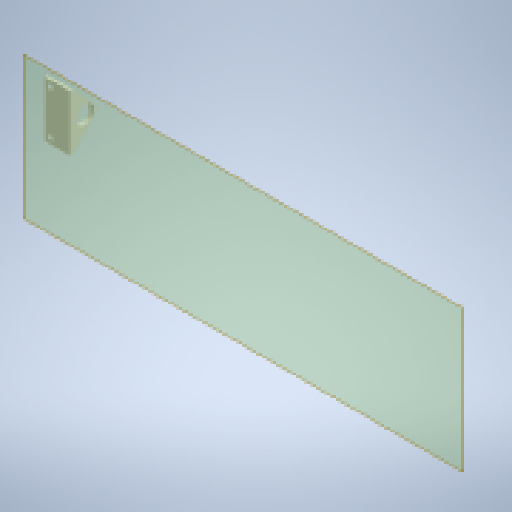
# Autodesk Inventor part: tumbler_holder
Saved by Autodesk Inventor 2024 (Build 280153000, 153)
## iProperties
Created: 2026-03-17
Part Number: tumbler_holder
Material: Generic
Document SubType Name: Modeling
Designer: SEMEN
Density: 1 g/cm^3
Appearance: Default
Author: SEMEN
Autodesk Inventor part; units mm, degrees
ref_plane "YZ Plane" through (0, 0, 0) normal (1, 0, 0) x (0, 1, 0)
ref_plane "XZ Plane" through (0, 0, 0) normal (0, 1, 0) x (-1, 0, 0)
ref_plane "XY Plane" through (0, 0, 0) normal (0, 0, 1) x (1, 0, 0)
ref_plane "Work Plane1" through (-14.6708, -27.7298, 48.581) normal (0, 0, -1) x (-1, 0, 0)
sketch "Sketch1" plane through (-14.6708, -27.7298, 48.581) normal (0, 0, -1) x (-1, 0, 0)
  circle A0 centre (26, 15.5) radius 3.3 projected
  circle A1 centre (26, -14) radius 3.3 projected
  line L0 (12.7, 19.5) -> (30, 19.5)
  line L1 (30, 19.5) -> (30, -18)
  line L2 (30, -18) -> (12.7, -18)
  line L3 (12.7, -18) -> (12.7, 19.5)
  line L4 (15.7, 19.5) -> (15.7, -18)
  point P0 (-14.6708, 27.7298)
  dimension "d0" = 4
  dimension "d1" = 4
  dimension "d2" = 4
  dimension "d3" = 10
  dimension "d4" = 3
  constraints: 10 end point, 2 parallel, 2 perpendicular, 2 point on line, 1 horizontal
  measures "d0" distance from line of L1 A0.centre
  measures "d1" distance from line of L0 A0.centre
  measures "d2" distance from line of L2 A1.centre
  measures "d3" distance edge to line of A0 L3
  measures "d4" distance between parallel lines of L3 L4
extrude "Extrusion1" add sketch "Sketch1" along normal blind 2 contours A0 | A1 | L0 L4 L2 L3 | L0 L1 L2 L4
sketch "Sketch2" plane through (-14.6708, -27.7298, 46.581) normal (0, 0, -1) x (-1, 0, 0)
  line L0 (15.7, 19.5) -> (15.7, -18) projected
  line L1 (12.7, 19.5) -> (12.7, -18) projected
  circle A0 centre (26, 15.5) radius 3.3 projected
  circle A1 centre (26, -14) radius 3.3 projected
  line L2 (30, 19.5) -> (12.7, 19.5) projected
  line L3 (12.7, -18) -> (30, -18) projected
  point P0 (-14.6708, 27.7298)
hole "Hole1" at (-40.6708, -12.2298, 46.581) at (-40.6708, -41.7298, 46.581) direction (0, 0, 1) diameter 3.4 end through all countersink diameter 6.6 countersink angle 90 clearance for "Countersunk Head GOST 12876-67" size "M3" standard "GOST"
sketch "Sketch3" plane through (-14.6708, -27.7298, 46.581) normal (0, 0, -1) x (-1, 0, 0)
  line L0 (30, 19.5) -> (12.7, 19.5) projected
  line L1 (12.7, 19.5) -> (12.7, -18) projected
  line L2 (15.7, 19.5) -> (15.7, -18) projected
  line L3 (12.7, -18) -> (30, -18) projected
  point P0 (-14.6708, 27.7298)
extrude "Extrusion2" add sketch "Sketch3" along normal blind 62.25
sketch "Sketch4" plane through (-30.3708, -45.7298, 46.581) normal (-1, 0, 0) x (0, 0, 1)
  line L0 (2, 0) -> (-62.25, 0) projected
  line L1 (-8, 0) -> (-8, 37.5) construction
  line L2 (0, 37.5) -> (-62.25, 37.5) projected
  circle A0 centre (-8, 18.75) radius 7
  line L3 (0, 37.5) -> (0, 0) projected
  circle A1 centre (-8, 18.75) radius 6
  line L4 (0, 0) -> (-13.1037, 13.9591)
  line L5 (-13.1037, 23.5409) -> (0, 37.5)
  line L6 (-62.25, 0) -> (-62.25, 37.5) projected
  point P0 (-46.581, 45.7298)
  dimension "d16" = 14
  dimension "d17" = 8
  dimension "d18" = 12
  constraints: 6 end point, 2 centre point, 2 point on circle, 2 point on line, 2 tangent, 1 coincident, 1 midpoint, 1 vertical
  measures "d16" diameter of A0
  measures "d17" distance between parallel lines of L3 L1
  measures "d18" diameter of A1
extrude "Extrusion3" cut sketch "Sketch4" against normal through all contours L0 L6 L2 L5 A0 L4 | A1
body "Solid1"
